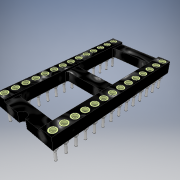
# Autodesk Inventor part: DIL28-Socket-Wide
Saved by Autodesk Inventor 2018 (Build 220112000, 112)
## iProperties
Created: 2020-04-18
Part Number: DIL28-Socket-Wide
Material: Všeobecné
Document SubType Name: Modeling
Designer: Jozko Mrkvicka
Density: 1 g/cm^3
Appearance: Výchozí
Author: Jozko Mrkvicka
Autodesk Inventor part; units mm, degrees
ref_plane "YZ Plane" through (0, 0, 0) normal (1, 0, 0) x (0, 1, 0)
ref_plane "XZ Plane" through (0, 0, 0) normal (0, 1, 0) x (-1, 0, 0)
ref_plane "XY Plane" through (0, 0, 0) normal (0, 0, 1) x (1, 0, 0)
sketch "Náčrt1" plane through (0, 0, 0) normal (0, 1, 0) x (-1, 0, 0)
  line L0 (17.78, 0) -> (17.78, -35.56)
  line L1 (17.78, -35.56) -> (0, -35.56)
  line L2 (0, -35.56) -> (0, 0)
  line L3 (0, 0) -> (3.175, 0)
  line L4 (3.175, -35.56) -> (0, -35.56)
  line L5 (0, -35.56) -> (0, 0)
  line L6 (17.78, 0) -> (14.605, 0)
  line L7 (6.985, -35.56) -> (17.78, -35.56)
  line L8 (17.78, -35.56) -> (17.78, 0)
  line L9 (3.81, -3.175) -> (13.97, -3.175)
  line L10 (6.985, -35.56) -> (3.175, -35.56)
  line L11 (3.81, -32.385) -> (13.97, -32.385)
  line L12 (3.81, -16.1925) -> (13.97, -16.1925)
  line L13 (13.97, -19.3675) -> (3.81, -19.3675)
  line L14 (14.605, -3.81) -> (14.605, -15.5575)
  line L15 (14.605, -20.0025) -> (14.605, -31.75)
  line L16 (3.175, -3.81) -> (3.175, -15.5575)
  line L17 (3.175, -20.0025) -> (3.175, -31.75)
  arc A0 (7.62, 0) -> (10.16, 0) centre (8.89, 0) ccw
  line L18 (0, 0) -> (7.62, 0)
  line L19 (10.16, 0) -> (17.78, 0)
  line L20 (14.605, 0) -> (10.16, 0)
  line L21 (7.62, 0) -> (3.175, 0)
  arc A1 (14.605, -3.81) -> (13.97, -3.175) centre (13.97, -3.81) ccw
  arc A2 (3.81, -3.175) -> (3.175, -3.81) centre (3.81, -3.81) ccw
  arc A3 (3.175, -15.5575) -> (3.81, -16.1925) centre (3.81, -15.5575) ccw
  arc A4 (13.97, -16.1925) -> (14.605, -15.5575) centre (13.97, -15.5575) ccw
  arc A5 (14.605, -20.0025) -> (13.97, -19.3675) centre (13.97, -20.0025) ccw
  arc A6 (3.81, -19.3675) -> (3.175, -20.0025) centre (3.81, -20.0025) ccw
  arc A7 (13.97, -32.385) -> (14.605, -31.75) centre (13.97, -31.75) ccw
  arc A8 (3.175, -31.75) -> (3.81, -32.385) centre (3.81, -31.75) ccw
  dimension "d0" = 17.78
  dimension "d1" = 35.56
  dimension "d6" = 2.54
  constraints: 44 end point, 18 point on circle, 16 tangent, 13 parallel, 9 centre point, 8 horizontal, 7 equal radius, 6 perpendicular, 2 point on line
  measures "d0" distance of L0.end L1.end
  measures "d1" distance of L0.start L0.end
  measures "d6" diameter of A0
extrude "Vysunutí8" add sketch "Náčrt1" along normal blind 3.175
sketch "Náčrt8" plane through (0, 3.175, 0) normal (0, 1, 0) x (1, 0, 0)
  line L0 (-14.605, 36.0555) -> (-3.175, 36.0555)
  line L1 (-3.175, 36.0555) -> (-3.175, -1.5875)
  line L2 (-3.175, -1.5875) -> (-14.605, -1.5875)
  line L3 (-14.605, -1.5875) -> (-14.605, 36.0555)
  point P0 (0, 0)
  constraints: 8 end point, 2 parallel, 1 horizontal, 1 perpendicular
extrude "Vysunutí9" cut sketch "Náčrt8" against normal blind 0.635
sketch "Náčrt9" plane through (0, 3.175, 0) normal (0, 1, 0) x (1, 0, 0)
  circle A0 centre (-1.27, 1.27) radius 0.635
  circle A1 centre (-1.27, 26.67) radius 0.635
  circle A2 centre (-1.27, 31.75) radius 0.635
  circle A3 centre (-1.27, 21.59) radius 0.635
  circle A4 centre (-1.27, 16.51) radius 0.635
  circle A5 centre (-1.27, 11.43) radius 0.635
  circle A6 centre (-1.27, 6.35) radius 0.635
  circle A7 centre (-1.27, 1.27) radius 0.635
  circle A8 centre (-1.27, 3.81) radius 0.635
  circle A9 centre (-1.27, 8.89) radius 0.635
  circle A10 centre (-1.27, 13.97) radius 0.635
  circle A11 centre (-1.27, 19.05) radius 0.635
  circle A12 centre (-1.27, 34.29) radius 0.635
  circle A13 centre (-1.27, 29.21) radius 0.635
  circle A14 centre (-1.27, 24.13) radius 0.635
  circle A15 centre (-16.51, 11.43) radius 0.635
  circle A16 centre (-16.51, 16.51) radius 0.635
  circle A17 centre (-16.51, 21.59) radius 0.635
  circle A18 centre (-16.51, 26.67) radius 0.635
  circle A19 centre (-16.51, 31.75) radius 0.635
  circle A20 centre (-16.51, 8.89) radius 0.635
  circle A21 centre (-16.51, 3.81) radius 0.635
  circle A22 centre (-16.51, 1.27) radius 0.635
  circle A23 centre (-16.51, 6.35) radius 0.635
  circle A24 centre (-16.51, 34.29) radius 0.635
  circle A25 centre (-16.51, 29.21) radius 0.635
  circle A26 centre (-16.51, 24.13) radius 0.635
  circle A27 centre (-16.51, 19.05) radius 0.635
  circle A28 centre (-16.51, 13.97) radius 0.635
  point P0 (0, 0)
  point P1 (-16.51, 1.27)
  constraints: 29 centre point
extrude "Vysunutí10" cut sketch "Náčrt9" against normal blind 0.635
sketch "Náčrt11" plane through (-1.27, 2.54, -1.27) normal (0, 1, 0) x (1, 0, 0)
  circle A0 centre (0, 33.02) radius 0.3175
  circle A1 centre (0, 33.02) radius 0.3175
  circle A2 centre (0, 30.4778) radius 0.3153
  circle A3 centre (0, 27.94) radius 0.3175
  circle A4 centre (0, 27.94) radius 0.3175
  circle A5 centre (0, 25.4) radius 0.3175
  circle A6 centre (0, 25.4) radius 0.3175
  circle A7 centre (0, 22.86) radius 0.3175
  circle A8 centre (0, 22.86) radius 0.3175
  circle A9 centre (0, 20.32) radius 0.3175
  circle A10 centre (0, 20.32) radius 0.3175
  circle A11 centre (0, 17.78) radius 0.3175
  circle A12 centre (0, 17.78) radius 0.3175
  circle A13 centre (0, 15.24) radius 0.3175
  circle A14 centre (0, 15.24) radius 0.3175
  circle A15 centre (0, 12.7) radius 0.3175
  circle A16 centre (0, 12.7) radius 0.3175
  circle A17 centre (0, 10.16) radius 0.3175
  circle A18 centre (0, 10.16) radius 0.3175
  circle A19 centre (0, 7.62) radius 0.3175
  circle A20 centre (0, 5.08) radius 0.3175
  circle A21 centre (0, 5.08) radius 0.3175
  circle A22 centre (0, 2.54) radius 0.3175
  circle A23 centre (0, 0) radius 0.3175
  circle A24 centre (0, 0) radius 0.3175
  circle A25 centre (-15.24, 0) radius 0.3175
  circle A26 centre (-15.24, 0) radius 0.3175
  circle A27 centre (-15.24, 2.54) radius 0.3175
  circle A28 centre (-15.24, 5.08) radius 0.3175
  circle A29 centre (-15.24, 7.62) radius 0.3175
  circle A30 centre (-15.24, 7.62) radius 0.3175
  circle A31 centre (-15.24, 10.16) radius 0.3175
  circle A32 centre (-15.24, 10.16) radius 0.3175
  circle A33 centre (-15.24, 12.7) radius 0.3175
  circle A34 centre (-15.24, 15.24) radius 0.3175
  circle A35 centre (-15.24, 15.24) radius 0.3175
  circle A36 centre (-15.24, 17.78) radius 0.3175
  circle A37 centre (-15.24, 17.78) radius 0.3175
  circle A38 centre (-15.24, 20.32) radius 0.3175
  circle A39 centre (-15.24, 22.86) radius 0.3175
  circle A40 centre (-15.24, 22.86) radius 0.3175
  circle A41 centre (-15.24, 25.4) radius 0.3175
  circle A42 centre (-15.24, 27.94) radius 0.3175
  circle A43 centre (-15.24, 30.48) radius 0.3175
  circle A44 centre (-15.24, 33.02) radius 0.3175
  circle A45 centre (-15.24, 0) radius 0.635 projected
  point P0 (1.27, -1.27)
  point P1 (1.27, 1.27)
  constraints: 45 centre point, 24 coincident
extrude "Vysunutí11" cut sketch "Náčrt11" against normal blind 1.27 contours A0 | A2 | A3 | A5 | A7 | A9 | A11 | A13 | A15 | A17 | A19 | A20 | A22 | A23 | A25 | A27 | A28 | A29 | A31 | A33 | A34 | A36 | A38 | A39 | A41 | A42 | A43 | A44
sketch "Náčrt12" plane through (0, 3.175, 0) normal (0, 1, 0) x (1, 0, 0)
  circle A0 centre (-16.5029, 1.27) radius 0.9525
  circle A1 centre (-16.5029, 8.89) radius 0.9525
  circle A2 centre (-16.5029, 3.81) radius 0.9525
  circle A3 centre (-16.5029, 6.35) radius 0.9525
  circle A4 centre (-16.5029, 11.43) radius 0.9525
  circle A5 centre (-16.5029, 13.97) radius 0.9525
  circle A6 centre (-16.5029, 16.51) radius 0.9525
  circle A7 centre (-16.5029, 19.05) radius 0.9525
  circle A8 centre (-16.5029, 21.59) radius 0.9525
  circle A9 centre (-16.5029, 24.13) radius 0.9525
  circle A10 centre (-16.5029, 26.67) radius 0.9525
  circle A11 centre (-16.5029, 29.21) radius 0.9525
  circle A12 centre (-16.5029, 31.75) radius 0.9525
  circle A13 centre (-16.5029, 34.29) radius 0.9525
  circle A14 centre (-1.27, 1.27) radius 0.9525
  circle A15 centre (-1.27, 3.81) radius 0.9525
  circle A16 centre (-1.27, 6.35) radius 0.9525
  circle A17 centre (-1.27, 8.89) radius 0.9525
  circle A18 centre (-1.27, 11.43) radius 0.9525
  circle A19 centre (-1.27, 13.97) radius 0.9525
  circle A20 centre (-1.27, 16.51) radius 0.9525
  circle A21 centre (-1.27, 19.05) radius 0.9525
  circle A22 centre (-1.27, 21.59) radius 0.9525
  circle A23 centre (-1.27, 24.13) radius 0.9525
  circle A24 centre (-1.27, 26.67) radius 0.9525
  circle A25 centre (-1.27, 29.21) radius 0.9525
  circle A26 centre (-1.27, 31.75) radius 0.9525
  circle A27 centre (-1.27, 34.29) radius 0.9525
  point P0 (0, 0)
  point P1 (-16.5029, 1.27)
  constraints: 28 centre point
extrude "Vysunutí12" cut sketch "Náčrt12" against normal blind 0.0254
sketch "Náčrt13" plane through (0, 0, 0) normal (0, -1, 0) x (1, 0, 0)
  circle A0 centre (-16.51, -1.27) radius 0.635 projected
  circle A1 centre (-16.51, -3.81) radius 0.635 projected
  circle A2 centre (-16.51, -6.35) radius 0.635 projected
  circle A3 centre (-16.51, -8.89) radius 0.635 projected
  circle A4 centre (-16.51, -11.43) radius 0.635 projected
  circle A5 centre (-16.51, -13.97) radius 0.635 projected
  circle A6 centre (-16.51, -16.51) radius 0.635 projected
  circle A7 centre (-16.51, -19.05) radius 0.635 projected
  circle A8 centre (-16.51, -21.59) radius 0.635 projected
  circle A9 centre (-16.51, -24.13) radius 0.635 projected
  circle A10 centre (-16.51, -26.67) radius 0.635 projected
  circle A11 centre (-16.51, -29.21) radius 0.635 projected
  circle A12 centre (-16.51, -31.75) radius 0.635 projected
  circle A13 centre (-16.51, -34.29) radius 0.635 projected
  circle A14 centre (-1.27, -34.29) radius 0.635 projected
  circle A15 centre (-1.27, -31.75) radius 0.635 projected
  circle A16 centre (-1.27, -29.21) radius 0.635 projected
  circle A17 centre (-1.27, -26.67) radius 0.635 projected
  circle A18 centre (-1.27, -24.13) radius 0.635 projected
  circle A19 centre (-1.27, -21.59) radius 0.635 projected
  circle A20 centre (-1.27, -19.05) radius 0.635 projected
  circle A21 centre (-1.27, -16.51) radius 0.635 projected
  circle A22 centre (-1.27, -13.97) radius 0.635 projected
  circle A23 centre (-1.27, -11.43) radius 0.635 projected
  circle A24 centre (-1.27, -8.89) radius 0.635 projected
  circle A25 centre (-1.27, -6.35) radius 0.635 projected
  circle A26 centre (-1.27, -3.81) radius 0.635 projected
  circle A27 centre (-1.27, -1.27) radius 0.635 projected
  point P0 (0, 0)
extrude "Vysunutí13" add sketch "Náčrt13" along normal blind 1.905
chamfer "Zkosení29" distance 0.3175 distance2 0.635 1 edges at (-1.905, -1.905, -1.27) measured on face at (-1.0935, -1.905, -1.2787)
chamfer "Zkosení30" distance 0.3175 distance2 0.635 1 edges at (-1.905, -1.905, -3.81) measured on face at (-1.2445, -1.905, -4.0201)
chamfer "Zkosení31" distance 0.3175 distance2 0.635 1 edges at (-1.905, -1.905, -6.35) measured on face at (-1.0645, -1.905, -6.4007)
chamfer "Zkosení32" distance 0.3175 distance2 0.635 1 edges at (-1.905, -1.905, -8.89) measured on face at (-1.4636, -1.905, -8.9377)
chamfer "Zkosení33" distance 0.3175 distance2 0.635 1 edges at (-1.905, -1.905, -11.43) measured on face at (-1.4636, -1.905, -11.4777)
chamfer "Zkosení34" distance 0.3175 distance2 0.635 1 edges at (-1.905, -1.905, -13.97) measured on face at (-1.4636, -1.905, -14.0177)
chamfer "Zkosení35" distance 0.3175 distance2 0.635 1 edges at (-1.905, -1.905, -16.51) measured on face at (-1.0826, -1.905, -16.5129)
chamfer "Zkosení36" distance 0.3175 distance2 0.635 1 edges at (-1.905, -1.905, -19.05) measured on face at (-1.0826, -1.905, -19.0529)
chamfer "Zkosení37" distance 0.3175 distance2 0.635 1 edges at (-1.905, -1.905, -21.59) measured on face at (-1.0826, -1.905, -21.5929)
chamfer "Zkosení38" distance 0.3175 distance2 0.635 1 edges at (-1.905, -1.905, -24.13) measured on face at (-1.0826, -1.905, -24.1329)
chamfer "Zkosení39" distance 0.3175 distance2 0.635 1 edges at (-1.905, -1.905, -26.67) measured on face at (-1.0826, -1.905, -26.6729)
chamfer "Zkosení40" distance 0.3175 distance2 0.635 1 edges at (-1.905, -1.905, -29.21) measured on face at (-1.0826, -1.905, -29.2129)
chamfer "Zkosení41" distance 0.3175 distance2 0.635 1 edges at (-17.145, -1.905, -34.29) measured on face at (-16.5355, -1.905, -34.0799)
chamfer "Zkosení42" distance 0.3175 distance2 0.635 1 edges at (-17.145, -1.905, -31.75) measured on face at (-16.4845, -1.905, -31.9357)
chamfer "Zkosení43" distance 0.3175 distance2 0.635 1 edges at (-17.145, -1.905, -29.21) measured on face at (-16.6813, -1.905, -29.3842)
chamfer "Zkosení44" distance 0.3175 distance2 0.635 1 edges at (-17.145, -1.905, -26.67) measured on face at (-16.6813, -1.905, -26.8442)
chamfer "Zkosení45" distance 0.3175 distance2 0.635 1 edges at (-17.145, -1.905, -24.13) measured on face at (-16.917, -1.905, -24.1537)
chamfer "Zkosení46" distance 0.3175 distance2 0.635 1 edges at (-17.145, -1.905, -21.59) measured on face at (-16.6813, -1.905, -21.7642)
chamfer "Zkosení47" distance 0.3175 distance2 0.635 1 edges at (-17.145, -1.905, -19.05) measured on face at (-16.917, -1.905, -19.0737)
chamfer "Zkosení48" distance 0.3175 distance2 0.635 1 edges at (-17.145, -1.905, -16.51) measured on face at (-16.3387, -1.905, -16.3358)
chamfer "Zkosení49" distance 0.3175 distance2 0.635 1 edges at (-17.145, -1.905, -13.97) measured on face at (-16.3387, -1.905, -13.7958)
chamfer "Zkosení50" distance 0.3175 distance2 0.635 1 edges at (-17.145, -1.905, -11.43) measured on face at (-16.3387, -1.905, -11.2558)
chamfer "Zkosení51" distance 0.3175 distance2 0.635 1 edges at (-17.145, -1.905, -8.89) measured on face at (-16.3387, -1.905, -8.7158)
chamfer "Zkosení52" distance 0.3175 distance2 0.635 1 edges at (-17.145, -1.905, -6.35) measured on face at (-16.917, -1.905, -6.3737)
chamfer "Zkosení53" distance 0.3175 distance2 0.635 1 edges at (-17.145, -1.905, -3.81) measured on face at (-16.917, -1.905, -3.8337)
chamfer "Zkosení54" distance 0.3175 distance2 0.635 1 edges at (-17.145, -1.905, -1.27) measured on face at (-16.917, -1.905, -1.2937)
chamfer "Zkosení55" distance 0.3175 distance2 0.635 1 edges at (-1.905, -1.905, -31.75) measured on face at (-1.2445, -1.905, -31.9357)
chamfer "Zkosení56" distance 0.3175 distance2 0.635 1 edges at (-1.905, -1.905, -34.29) measured on face at (-1.3451, -1.905, -34.0921)
sketch "Náčrt14" plane through (-1.27, -1.905, -1.27) normal (0, -1, 0) x (1, 0, 0)
  circle A0 centre (0, 0) radius 0.3175 projected
  circle A1 centre (0, -2.54) radius 0.3175 projected
  circle A2 centre (0, -5.08) radius 0.3175 projected
  circle A3 centre (0, -7.62) radius 0.3175 projected
  circle A4 centre (0, -10.16) radius 0.3175 projected
  circle A5 centre (0, -12.7) radius 0.3175 projected
  circle A6 centre (0, -15.24) radius 0.3175 projected
  circle A7 centre (0, -17.78) radius 0.3175 projected
  circle A8 centre (0, -20.32) radius 0.3175 projected
  circle A9 centre (0, -22.86) radius 0.3175 projected
  circle A10 centre (0, -25.4) radius 0.3175 projected
  circle A11 centre (0, -27.94) radius 0.3175 projected
  circle A12 centre (0, -30.4778) radius 0.3153 projected
  circle A13 centre (0, -33.02) radius 0.3175 projected
  circle A14 centre (-15.24, -33.02) radius 0.3175 projected
  circle A15 centre (-15.24, -30.48) radius 0.3175 projected
  circle A16 centre (-15.24, -27.94) radius 0.3175 projected
  circle A17 centre (-15.24, -25.4) radius 0.3175 projected
  circle A18 centre (-15.24, -22.86) radius 0.3175 projected
  circle A19 centre (-15.24, -20.32) radius 0.3175 projected
  circle A20 centre (-15.24, -17.78) radius 0.3175 projected
  circle A21 centre (-15.24, -15.24) radius 0.3175 projected
  circle A22 centre (-15.24, -12.7) radius 0.3175 projected
  circle A23 centre (-15.24, -10.16) radius 0.3175 projected
  circle A24 centre (-15.24, -7.62) radius 0.3175 projected
  circle A25 centre (-15.24, -5.08) radius 0.3175 projected
  circle A26 centre (-15.24, -2.54) radius 0.3175 projected
  circle A27 centre (-15.24, 0) radius 0.3175 projected
  point P0 (1.27, 1.27)
extrude "Vysunutí14" add sketch "Náčrt14" along normal blind 2.54
fillet "Zaoblení2" radius 0.127 28 edges at (-16.8275, -4.445, -1.27) (-16.8275, -4.445, -3.81) (-16.8275, -4.445, -6.35) (-16.8275, -4.445, -8.89) (-16.8275, -4.445, -11.43) (-16.8275, -4.445, -13.97) (-16.8275, -4.445, -16.51) (-16.8275, -4.445, -19.05) (-16.8275, -4.445, -21.59) (-16.8275, -4.445, -24.13) (-16.8275, -4.445, -26.67) (-16.8275, -4.445, -29.21) (-16.8275, -4.445, -31.75) (-16.8275, -4.445, -34.29) (-1.5875, -4.445, -34.29) (-1.5853, -4.445, -31.7478) (-1.5875, -4.445, -29.21) (-1.5875, -4.445, -26.67) (-1.5875, -4.445, -24.13) (-1.5875, -4.445, -21.59) (-1.5875, -4.445, -19.05) (-1.5875, -4.445, -16.51) (-1.5875, -4.445, -13.97) (-1.5875, -4.445, -11.43) (-1.5875, -4.445, -8.89) (-1.5875, -4.445, -6.35) (-1.5875, -4.445, -3.81) (-1.5875, -4.445, -1.27)
